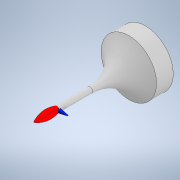
# Autodesk Inventor part: EndEffector
Saved by Autodesk Inventor 2021 (Build 250183000, 183)
## iProperties
Created: 2024-09-30
Part Number: EndEffector
Material: Generic
Document SubType Name: Modeling
Designer: Swoby
Density: 1 g/cm^3
Appearance: Default
Author: Swoby
Autodesk Inventor part; units mm, degrees
sketch "Sketch1" plane through (0, 0, 0) normal (1, 0, 0) x (0, 1, 0)
  line L0 (0, 0) -> (0, 80)
  line L1 (0, 0) -> (25, 0)
  line L2 (25, 0) -> (25, 15)
  line L3 (25, 15) -> (2.5, 15) construction
  line L4 (2.5, 15) -> (2.5, 50) construction
  line L5 (2.5, 80) -> (0, 80)
  arc A0 (2.5, 50) -> (25, 15) centre (40.9722, 50) ccw
  line L6 (2.5, 50) -> (2.5, 80)
  dimension "d0" = 50
  dimension "d1" = 80
  dimension "d2" = 15
  dimension "d3" = 5
  dimension "d4" = 35
  constraints: 14 end point, 4 perpendicular, 2 point on circle, 2 tangent, 1 centre point, 1 horizontal, 1 vertical
  measures "d0" diameter of L2 L0
  measures "d1" distance between parallel lines of L1 L5
  measures "d2" distance of L1.end L2.end
  measures "d3" diameter of L4 L0
  measures "d4" vertical distance of L2.end L4.end
revolve "Revolution1" add sketch "Sketch1" angle 360 about axis through (0, 0, 0) along (0, 0, 1)
ref_plane "Work Plane1" through (0, 0, 100) normal (0, 0, 1) x (1, 0, 0)
sketch "Sketch3" plane through (0, 0, 100) normal (0, 0, 1) x (1, 0, 0)
  line L0 (-0.5, -0.5) -> (0.5, -0.5)
  line L1 (0.5, -0.5) -> (0.5, 0.5)
  line L2 (0.5, 0.5) -> (-0.5, 0.5)
  line L3 (-0.5, 0.5) -> (-0.5, -0.5)
  line L4 (-0.5, -0.5) -> (0.5, 0.5) construction
  line L5 (0.5, -0.5) -> (-0.5, 0.5) construction
  point P0 (0, 0)
  dimension "d7" = 1
  dimension "d8" = 1
  constraints: 12 end point, 2 midpoint, 2 parallel, 1 horizontal, 1 perpendicular
  measures "d7" distance of L2.end L1.end
  measures "d8" distance of L0.end L1.end
ref_plane "Work Plane2" through (0, 0, 90) normal (0, 0, 1) x (1, 0, 0)
sketch "Sketch4" plane through (0, 0, 90) normal (0, 0, 1) x (1, 0, 0)
  line L0 (-2.5, -2.5) -> (2.5, -2.5)
  line L1 (2.5, -2.5) -> (2.5, 2.5)
  line L2 (2.5, 2.5) -> (-2.5, 2.5)
  line L3 (-2.5, 2.5) -> (-2.5, -2.5)
  line L4 (-2.5, -2.5) -> (2.5, 2.5) construction
  line L5 (2.5, -2.5) -> (-2.5, 2.5) construction
  point P0 (0, 0)
  dimension "d10" = 5
  dimension "d11" = 5
  constraints: 12 end point, 2 midpoint, 2 parallel, 1 horizontal, 1 perpendicular
  measures "d10" distance of L2.end L1.end
  measures "d11" distance of L1.end L0.end
loft "Loft1" add profiles "Sketch4", "Sketch3" section 1 edges at (0, -2.5, 80)
sketch "Sketch5" plane through (0, 0, 0) normal (1, 0, 0) x (0, 1, 0)
  line L0 (1.7678, 80) -> (1.7678, 80) projected
  line L1 (1.7678, 80) -> (-1.7678, 80) projected
  line L2 (-1.7678, 80) -> (-1.7678, 80) projected
  line L3 (-1.7678, 80) -> (1.7678, 80) projected
  line L4 (-2.5, 50) -> (2.5, 50) projected
  line L5 (-1.5, 81.5) -> (1.5, 81.5)
  line L6 (1.5, 81.5) -> (1.5, 78.5)
  line L7 (1.5, 78.5) -> (-1.5, 78.5)
  line L8 (-1.5, 78.5) -> (-1.5, 81.5)
  line L9 (-1.7678, 80) -> (1.7678, 80) projected
  line L10 (-1.5, 81.5) -> (1.5, 78.5) construction
  line L11 (1.5, 81.5) -> (-1.5, 78.5) construction
  point P0 (0, 0)
  point P1 (0, 80)
  dimension "d18" = 3
  dimension "d19" = 3
  constraints: 12 end point, 3 midpoint, 2 parallel, 1 horizontal, 1 perpendicular
  measures "d18" distance of L6.end L7.end
  measures "d19" distance of L5.end L6.end
ref_plane "Work Plane3" through (10, 0, 0) normal (1, 0, 0) x (0, 1, 0)
sketch "Sketch6" plane through (10, 0, 0) normal (1, 0, 0) x (0, 1, 0)
  line L0 (1.7678, 80) -> (1.7678, 80) projected
  line L1 (1.7678, 80) -> (-2.5, 80) projected
  line L2 (-2.5, 80) -> (-1.7678, 80) projected
  line L3 (-1.7678, 80) -> (1.7678, 80) projected
  line L4 (-2.5, 50) -> (2.5, 50) projected
  line L5 (-0.25, 80.25) -> (0.25, 80.25)
  line L6 (0.25, 80.25) -> (0.25, 79.75)
  line L7 (0.25, 79.75) -> (-0.25, 79.75)
  line L8 (-0.25, 79.75) -> (-0.25, 80.25)
  line L9 (-2.5, 80) -> (1.7678, 80) projected
  line L10 (-0.25, 80.25) -> (0.25, 79.75) construction
  line L11 (0.25, 80.25) -> (-0.25, 79.75) construction
  point P0 (0, 0)
  point P1 (0, 80)
  dimension "d21" = 0.5
  dimension "d22" = 0.5
  constraints: 12 end point, 2 midpoint, 2 parallel, 1 horizontal, 1 perpendicular, 1 point on line
  measures "d21" distance of L6.end L7.end
  measures "d22" distance of L5.end L6.end
loft "Loft2" add profiles "Sketch5", "Sketch6"
body "Solid1"
